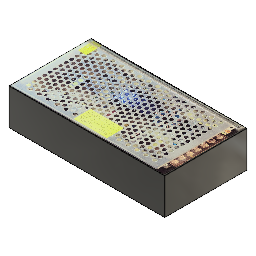
Full Assembly v14 (Autodesk Fusion 360 archive; units mm, degrees)
design "Power Supply"
Autodesk Fusion 360 part; units mm, degrees
(part 1 of 6)
sketch "Sketch1" plane through (0, 0, 0) normal (0, 0, 1) x (1, 0, 0)
  line L0 (0, 0) -> (214, 0)
  line L1 (214, 0) -> (214, 113)
  line L2 (214, 113) -> (0, 113)
  line L3 (0, 113) -> (0, 0)
  dimension "d1" = 214
  dimension "d2" = 113
  constraint horizontal L0
  constraint vertical L1
  constraint horizontal L2
  constraint vertical L3
  constraint coincident L0.start L3.end
  measures "d1" distance of L0.start L0.end
  measures "d2" distance of L0.start L2.end
extrude "Extrude1" add sketch "Sketch1" along normal blind 50

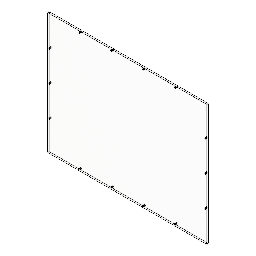
design "Front Acrylic"
Autodesk Fusion 360 part; units mm, degrees
sketch "Sketch1" plane through (0, 0, 0) normal (0, 1, 0) x (1, 0, 0)
  line L0 (0, 0) -> (635, 0)
  line L1 (635, 0) -> (635, -483.55)
  line L2 (635, -483.55) -> (0, -483.55)
  line L3 (0, -483.55) -> (0, 0)
  circle A0 centre (127, -477.05) radius 2.25
  circle A1 centre (254, -477.05) radius 2.25
  circle A2 centre (508, -477.05) radius 2.25
  circle A3 centre (381, -477.05) radius 2.25
  circle A4 centre (628.5, -362.775) radius 2.25
  circle A5 centre (628.5, -241.775) radius 2.25
  circle A6 centre (628.5, -120.775) radius 2.25
  circle A7 centre (6.5, -362.775) radius 2.25
  circle A8 centre (6.5, -241.775) radius 2.25
  circle A9 centre (6.5, -120.775) radius 2.25
  circle A10 centre (127, -6.5) radius 2.25
  circle A11 centre (254, -6.5) radius 2.25
  circle A12 centre (381, -6.5) radius 2.25
  circle A13 centre (508, -6.5) radius 2.25
  dimension "d1" = 483.55
  dimension "d2" = 635
  dimension "d5" = 6.5
  dimension "d6" = 6.5
  dimension "d7" = 127
  dimension "d8" = 127
  dimension "d9" = 127
  dimension "d10" = 127
  dimension "d11" = 6.5
  dimension "d12" = 6.5
  dimension "d13" = 6.5
  dimension "d14" = 6.5
  dimension "d15" = 6.5
  dimension "d18" = 121
  dimension "d19" = 4.5
  dimension "d21" = 121
  dimension "d22" = 121
  dimension "d23" = 6.5
  dimension "d24" = 6.5
  dimension "d26" = 6.5
  dimension "d27" = 127
  dimension "d28" = 127
  dimension "d29" = 127
  dimension "d30" = 127
  dimension "d31" = 6.5
  dimension "d32" = 6.5
  dimension "d33" = 6.5
  dimension "d34" = 6.5
  dimension "d53" = 241.775
  dimension "d54" = 121
  dimension "d55" = 241.775
  constraint horizontal L0
  constraint vertical L3
  constraint coincident L0.start L3.end
  constraint equal A0 A1
  constraint equal A1 A2
  constraint equal A2 A3
  constraint equal A3 A4
  constraint equal A4 A5
  constraint equal A5 A6
  constraint equal A0 A7
  constraint equal A7 A8
  constraint equal A8 A9
  constraint equal A10 A11
  constraint equal A11 A12
  constraint equal A12 A13
  constraint equal A9 A10
  constraint horizontal L2
  constraint vertical L1
  measures "d1" distance of L0.start L2.end
  measures "d2" distance of L0.start L0.end
  measures "d5" distance of L2 A0.centre
  measures "d6" distance of L2 A1.centre
  measures "d7" distance of L3 A0.centre
  measures "d8" distance of A0.centre A1.centre
  measures "d9" horizontal distance of A1.centre A3.centre
  measures "d10" horizontal distance of A2.centre A3.centre
  measures "d11" distance of L2 A3.centre
  measures "d12" distance of L2 A2.centre
  measures "d13" distance of L1 A4.centre
  measures "d14" distance of L1 A5.centre
  measures "d15" distance of L1 A6.centre
  measures "d18" distance of A5.centre A6.centre
  measures "d19" diameter of A0
  measures "d21" vertical distance of A7.centre A8.centre
  measures "d22" vertical distance of A8.centre A9.centre
  measures "d23" distance of L3 A7.centre
  measures "d24" distance of L3 A8.centre
  measures "d26" distance of L3 A9.centre
  measures "d27" horizontal distance of L0.start A10.centre
  measures "d28" distance of A10.centre A11.centre
  measures "d29" distance of A11.centre A12.centre
  measures "d30" distance of A12.centre A13.centre
  measures "d31" distance of L0 A10.centre
  measures "d32" distance of L0 A11.centre
  measures "d33" distance of L0 A12.centre
  measures "d34" distance of L0 A13.centre
  measures "d53" distance of L2 A5.centre
  measures "d54" distance of A4.centre A5.centre
  measures "d55" distance of L2 A8.centre
sketch "Sketch2" plane through (0, 0, 0) normal (0, 1, 0) x (1, 0, 0)
  line L0 (635, 0) -> (635, -483.55)
  line L1 (635, -483.55) -> (0, -483.55)
  line L2 (0, 0) -> (635, 0)
  line L3 (0, -483.55) -> (0, 0)
  line L4 (126, -8.5) -> (128, -8.5)
  arc A0 (128, -8.5) -> (128, -4.5) centre (128, -6.5) ccw
  line L5 (128, -4.5) -> (126, -4.5)
  arc A1 (126, -4.5) -> (126, -8.5) centre (126, -6.5) ccw
  line L6 (126, -6.5) -> (128, -6.5) construction
  line L7 (253, -8.5) -> (255, -8.5)
  arc A2 (255, -8.5) -> (255, -4.5) centre (255, -6.5) ccw
  line L8 (255, -4.5) -> (253, -4.5)
  arc A3 (253, -4.5) -> (253, -8.5) centre (253, -6.5) ccw
  line L9 (253, -6.5) -> (255, -6.5) construction
  line L10 (380, -8.5) -> (382, -8.5)
  arc A4 (382, -8.5) -> (382, -4.5) centre (382, -6.5) ccw
  line L11 (382, -4.5) -> (380, -4.5)
  arc A5 (380, -4.5) -> (380, -8.5) centre (380, -6.5) ccw
  line L12 (380, -6.5) -> (382, -6.5) construction
  line L13 (507, -8.5) -> (509, -8.5)
  arc A6 (509, -8.5) -> (509, -4.5) centre (509, -6.5) ccw
  line L14 (509, -4.5) -> (507, -4.5)
  arc A7 (507, -4.5) -> (507, -8.5) centre (507, -6.5) ccw
  line L15 (507, -6.5) -> (509, -6.5) construction
  line L16 (626.5, -119.775) -> (626.5, -121.775)
  arc A8 (626.5, -121.775) -> (630.5, -121.775) centre (628.5, -121.775) ccw
  line L17 (630.5, -121.775) -> (630.5, -119.775)
  arc A9 (630.5, -119.775) -> (626.5, -119.775) centre (628.5, -119.775) ccw
  line L18 (628.5, -119.775) -> (628.5, -121.775) construction
  line L19 (626.5, -240.775) -> (626.5, -242.775)
  arc A10 (626.5, -242.775) -> (630.5, -242.775) centre (628.5, -242.775) ccw
  line L20 (630.5, -242.775) -> (630.5, -240.775)
  arc A11 (630.5, -240.775) -> (626.5, -240.775) centre (628.5, -240.775) ccw
  line L21 (628.5, -240.775) -> (628.5, -242.775) construction
  line L22 (626.5, -361.775) -> (626.5, -363.775)
  arc A12 (626.5, -363.775) -> (630.5, -363.775) centre (628.5, -363.775) ccw
  line L23 (630.5, -363.775) -> (630.5, -361.775)
  arc A13 (630.5, -361.775) -> (626.5, -361.775) centre (628.5, -361.775) ccw
  line L24 (628.5, -361.775) -> (628.5, -363.775) construction
  line L25 (509, -475.05) -> (507, -475.05)
  arc A14 (507, -475.05) -> (507, -479.05) centre (507, -477.05) ccw
  line L26 (507, -479.05) -> (509, -479.05)
  arc A15 (509, -479.05) -> (509, -475.05) centre (509, -477.05) ccw
  line L27 (509, -477.05) -> (507, -477.05) construction
  line L28 (382, -475.05) -> (380, -475.05)
  arc A16 (380, -475.05) -> (380, -479.05) centre (380, -477.05) ccw
  line L29 (380, -479.05) -> (382, -479.05)
  arc A17 (382, -479.05) -> (382, -475.05) centre (382, -477.05) ccw
  line L30 (382, -477.05) -> (380, -477.05) construction
  line L31 (255, -475.05) -> (253, -475.05)
  arc A18 (253, -475.05) -> (253, -479.05) centre (253, -477.05) ccw
  line L32 (253, -479.05) -> (255, -479.05)
  arc A19 (255, -479.05) -> (255, -475.05) centre (255, -477.05) ccw
  line L33 (255, -477.05) -> (253, -477.05) construction
  line L34 (128, -475.05) -> (126, -475.05)
  arc A20 (126, -475.05) -> (126, -479.05) centre (126, -477.05) ccw
  line L35 (126, -479.05) -> (128, -479.05)
  arc A21 (128, -479.05) -> (128, -475.05) centre (128, -477.05) ccw
  line L36 (128, -477.05) -> (126, -477.05) construction
  line L37 (4.5, -361.775) -> (4.5, -363.775)
  arc A22 (4.5, -363.775) -> (8.5, -363.775) centre (6.5, -363.775) ccw
  line L38 (8.5, -363.775) -> (8.5, -361.775)
  arc A23 (8.5, -361.775) -> (4.5, -361.775) centre (6.5, -361.775) ccw
  line L39 (6.5, -361.775) -> (6.5, -363.775) construction
  line L40 (4.5, -240.775) -> (4.5, -242.775)
  arc A24 (4.5, -242.775) -> (8.5, -242.775) centre (6.5, -242.775) ccw
  line L41 (8.5, -242.775) -> (8.5, -240.775)
  arc A25 (8.5, -240.775) -> (4.5, -240.775) centre (6.5, -240.775) ccw
  line L42 (6.5, -240.775) -> (6.5, -242.775) construction
  line L43 (4.5, -119.775) -> (4.5, -121.775)
  arc A26 (4.5, -121.775) -> (8.5, -121.775) centre (6.5, -121.775) ccw
  line L44 (8.5, -121.775) -> (8.5, -119.775)
  arc A27 (8.5, -119.775) -> (4.5, -119.775) centre (6.5, -119.775) ccw
  line L45 (6.5, -119.775) -> (6.5, -121.775) construction
  point P0 (127, -6.5)
  point P1 (254, -6.5)
  point P2 (381, -6.5)
  point P3 (508, -6.5)
  point P4 (628.5, -120.775)
  point P5 (628.5, -241.775)
  point P6 (628.5, -362.775)
  point P7 (508, -477.05)
  point P8 (381, -477.05)
  point P9 (254, -477.05)
  point P10 (127, -477.05)
  point P11 (6.5, -362.775)
  point P12 (6.5, -241.775)
  point P13 (6.5, -120.775)
  point P14 (127, -6.5)
  point P15 (254, -6.5)
  point P16 (381, -6.5)
  point P17 (508, -6.5)
  point P18 (628.5, -120.775)
  point P19 (628.5, -241.775)
  point P20 (628.5, -362.775)
  point P21 (508, -477.05)
  point P22 (381, -477.05)
  point P23 (254, -477.05)
  point P24 (127, -477.05)
  point P25 (6.5, -362.775)
  point P26 (6.5, -241.775)
  point P27 (6.5, -120.775)
  point P28 (317.5, 0)
  dimension "d36" = 2
  dimension "d37" = 2
  dimension "d47" = 127
  dimension "d48" = 127
  dimension "d50" = 63.5
  dimension "d51" = 190.5
  dimension "d52" = 121
  constraint tangent L4 A0
  constraint tangent A0 L5
  constraint parallel L4 L5
  constraint tangent L5 A1
  constraint tangent L4 A1
  constraint horizontal L6
  constraint coincident P14 P0
  constraint midpoint L6 P14
  constraint tangent L7 A2
  constraint tangent A2 L8
  constraint parallel L7 L8
  constraint tangent L8 A3
  constraint tangent L7 A3
  constraint parallel L2 L9
  constraint coincident P15 P1
  constraint midpoint L9 P15
  constraint tangent L10 A4
  constraint tangent A4 L11
  constraint parallel L10 L11
  constraint tangent L11 A5
  constraint tangent L10 A5
  constraint parallel L2 L12
  constraint coincident P16 P2
  constraint midpoint L12 P16
  constraint tangent L13 A6
  constraint tangent A6 L14
  constraint parallel L13 L14
  constraint tangent L14 A7
  constraint tangent L13 A7
  constraint parallel L2 L15
  constraint coincident P17 P3
  constraint midpoint L15 P17
  constraint tangent L16 A8
  constraint tangent A8 L17
  constraint parallel L16 L17
  constraint tangent L17 A9
  constraint tangent L16 A9
  constraint perpendicular L13 L18
  constraint coincident P18 P4
  constraint midpoint L18 P18
  constraint tangent L19 A10
  constraint tangent A10 L20
  constraint parallel L19 L20
  constraint tangent L20 A11
  constraint tangent L19 A11
  constraint perpendicular L13 L21
  constraint coincident P19 P5
  constraint midpoint L21 P19
  constraint tangent L22 A12
  constraint tangent A12 L23
  constraint parallel L22 L23
  constraint tangent L23 A13
  constraint tangent L22 A13
  constraint parallel L19 L24
  constraint coincident P20 P6
  constraint midpoint L24 P20
  constraint tangent L25 A14
  constraint tangent A14 L26
  constraint parallel L25 L26
  constraint tangent L26 A15
  constraint tangent L25 A15
  constraint perpendicular L19 L27
  constraint coincident P21 P7
  constraint midpoint L27 P21
  constraint tangent L28 A16
  constraint tangent A16 L29
  constraint parallel L28 L29
  constraint tangent L29 A17
  constraint tangent L28 A17
  constraint parallel L1 L30
  constraint coincident P22 P8
  constraint midpoint L30 P22
  constraint tangent L31 A18
  constraint tangent A18 L32
  constraint parallel L31 L32
  constraint tangent L32 A19
  constraint tangent L31 A19
  constraint parallel L1 L33
  constraint coincident P23 P9
  constraint midpoint L33 P23
  constraint tangent L34 A20
  constraint tangent A20 L35
  constraint parallel L34 L35
  constraint tangent L35 A21
  constraint tangent L34 A21
  constraint parallel L1 L36
  constraint coincident P24 P10
  constraint midpoint L36 P24
  constraint tangent L37 A22
  constraint tangent A22 L38
  constraint parallel L37 L38
  constraint tangent L38 A23
  constraint tangent L37 A23
  constraint vertical L39
  constraint coincident P25 P11
  constraint midpoint L39 P25
  constraint tangent L40 A24
  constraint tangent A24 L41
  constraint parallel L40 L41
  constraint tangent L41 A25
  constraint tangent L40 A25
  constraint perpendicular L1 L42
  constraint coincident P26 P12
  constraint midpoint L42 P26
  constraint tangent L43 A26
  constraint tangent A26 L44
  constraint parallel L43 L44
  constraint tangent L44 A27
  constraint tangent L43 A27
  constraint parallel L3 L45
  constraint coincident P27 P13
  constraint midpoint L45 P27
  constraint equal A0 A3
  constraint equal L6 L9
  constraint equal A2 A5
  constraint equal L9 L12
  constraint equal A4 A7
  constraint equal L12 L15
  constraint equal A6 A9
  constraint equal L15 L18
  constraint equal A8 A11
  constraint equal L18 L21
  constraint equal L21 L24
  constraint equal A10 A13
  constraint equal A12 A15
  constraint equal L24 L27
  constraint equal A14 A17
  constraint equal L27 L30
  constraint equal A16 A19
  constraint equal L30 L33
  constraint equal A18 A21
  constraint equal L33 L36
  constraint equal A20 A22
  constraint equal L36 L39
  constraint equal A23 A24
  constraint equal L39 L42
  constraint equal A25 A26
  constraint equal L42 L45
  constraint midpoint L2 P28
  measures "d36" radius of A0
  measures "d37" distance of A1.centre A0.centre
  measures "d47" distance of P16 P17
  measures "d48" distance of P15 P16
  measures "d50" horizontal distance of P15 P28
  measures "d51" horizontal distance of P14 P28
  measures "d52" distance of P26 P27
sketch "Sketch3" plane through (0, 0, 0) normal (0, 1, 0) x (1, 0, 0)
  arc A0 (128, -8.5) -> (128, -4.5) centre (128, -6.5) ccw
  line L0 (126, -8.5) -> (128, -8.5)
  arc A1 (126, -4.5) -> (126, -8.5) centre (126, -6.5) ccw
  line L1 (128, -4.5) -> (126, -4.5)
  line L2 (116, -13) -> (138, -13)
  line L3 (138, -13) -> (138, 0)
  line L4 (138, 0) -> (116, 0)
  line L5 (116, 0) -> (116, -13)
  point P0 (126, -6.5)
  point P1 (127, -6.5)
  point P2 (128, -6.5)
  dimension "d42" = 10
  dimension "d43" = 10
  dimension "d44" = 6.5
  dimension "d45" = 6.5
  dimension "d46" = 6.5
  constraint horizontal L2
  constraint vertical L3
  constraint horizontal L4
  constraint vertical L5
  measures "d42" distance of P2 L3
  measures "d43" distance of P0 L5
  measures "d44" vertical distance of origin P1
  measures "d45" distance of P1 L4
  measures "d46" distance of P1 L2
extrude "Extrude2" add sketch "Sketch2" along normal blind 6.35
equation "d5 = ( 13 / 2 ) * 1 mm"
equation "d6 = d5"
equation "d7 = d2 / 5"
equation "d8 = d7"
equation "d9 = d8"
equation "d10 = d7"
equation "d11 = d5"
equation "d12 = d5"
equation "d13 = d5"
equation "d14 = d5"
equation "d15 = d5"
equation "d16 = d1 / 4"
equation "d18 = d54"
equation "d20 = d1 / 4"
equation "d21 = d54"
equation "d22 = d54"
equation "d23 = d5"
equation "d24 = d5"
equation "d26 = d5"
equation "d27 = d2 / 5"
equation "d28 = d27"
equation "d29 = d27"
equation "d30 = d27"
equation "d31 = d5"
equation "d32 = d5"
equation "d33 = d5"
equation "d34 = d5"
equation "d36 = ( 4 / 2 ) * 1 mm"
equation "d45 = d44"
equation "d46 = d44"
equation "d53 = d1 / 2"
equation "d55 = d1 / 2"

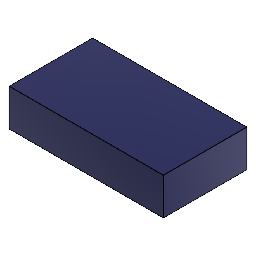
design "Power Distribution Board"
Autodesk Fusion 360 part; units mm, degrees
sketch "Sketch1" plane through (0, 0, 0) normal (0, 0, 1) x (1, 0, 0)
  line L0 (0, 0) -> (83.05, 0)
  line L1 (83.05, 0) -> (83.05, 44.95)
  line L2 (83.05, 44.95) -> (0, 44.95)
  line L3 (0, 44.95) -> (0, 0)
  dimension "d1" = 83.05
  dimension "d2" = 44.95
  constraint horizontal L0
  constraint vertical L1
  constraint horizontal L2
  constraint vertical L3
  constraint coincident L0.start L3.end
  measures "d1" distance of L0.start L0.end
  measures "d2" distance of L0.start L2.end
extrude "Extrude1" add sketch "Sketch1" along normal blind 20
equation "d1 = 82.55 mm + 0.5 mm"

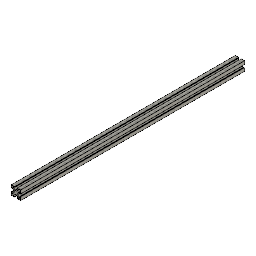
design "TS10-10"
Autodesk Fusion 360 part; units mm, degrees
sketch "Sketch1" plane through (0, 0, 0) normal (0, 1, 0) x (1, 0, 0)
  line L0 (0, 0) -> (0, 4.826)
  line L1 (0, 4.826) -> (2, 4.826)
  line L2 (2, 4.826) -> (7.874, 10.7)
  line L3 (7.874, 10.7) -> (3.302, 10.7)
  line L4 (3.302, 10.7) -> (3.302, 12.7)
  line L5 (3.302, 12.7) -> (12.7, 12.7)
  line L6 (12.7, 12.7) -> (12.7, 3.302)
  line L7 (12.7, 3.302) -> (10.7, 3.302)
  line L8 (10.7, 3.302) -> (10.7, 7.874)
  line L9 (10.7, 7.874) -> (4.826, 2)
  line L10 (4.826, 2) -> (4.826, 0)
  line L11 (4.826, 0) -> (0, 0)
  line L12 (0, 4.826) -> (-2, 4.826)
  line L13 (-4.826, 2) -> (-4.826, 0)
  line L14 (-7.874, 10.7) -> (-3.302, 10.7)
  line L15 (-10.7, 3.302) -> (-10.7, 7.874)
  line L16 (-4.826, 0) -> (0, 0)
  line L17 (-12.7, 3.302) -> (-10.7, 3.302)
  line L18 (-3.302, 10.7) -> (-3.302, 12.7)
  line L19 (-2, 4.826) -> (-7.874, 10.7)
  line L20 (-12.7, 12.7) -> (-12.7, 3.302)
  line L21 (-3.302, 12.7) -> (-12.7, 12.7)
  line L22 (-10.7, 7.874) -> (-4.826, 2)
  line L23 (0, -4.826) -> (2, -4.826)
  line L24 (12.7, -3.302) -> (10.7, -3.302)
  line L25 (7.874, -10.7) -> (3.302, -10.7)
  line L26 (3.302, -10.7) -> (3.302, -12.7)
  line L27 (3.302, -12.7) -> (12.7, -12.7)
  line L28 (-12.7, -3.302) -> (-10.7, -3.302)
  line L29 (10.7, -7.874) -> (4.826, -2)
  line L30 (-10.7, -7.874) -> (-4.826, -2)
  line L31 (-10.7, -3.302) -> (-10.7, -7.874)
  line L32 (-12.7, -12.7) -> (-12.7, -3.302)
  line L33 (12.7, -12.7) -> (12.7, -3.302)
  line L34 (4.826, -2) -> (4.826, 0)
  line L35 (2, -4.826) -> (7.874, -10.7)
  line L36 (10.7, -3.302) -> (10.7, -7.874)
  line L37 (0, -4.826) -> (-2, -4.826)
  line L38 (-7.874, -10.7) -> (-3.302, -10.7)
  line L39 (-4.826, -2) -> (-4.826, 0)
  line L40 (-3.302, -10.7) -> (-3.302, -12.7)
  line L41 (0, 0) -> (0, -4.826)
  line L42 (-2, -4.826) -> (-7.874, -10.7)
  line L43 (-3.302, -12.7) -> (-12.7, -12.7)
  dimension "d1" = 12.7
  dimension "d2" = 12.7
  dimension "d3" = 3.302
  dimension "d4" = 3.302
  dimension "d5" = 7.874
  dimension "d6" = 7.874
  dimension "d8" = 7.874
  dimension "d9" = 2
  dimension "d10" = 2
  constraint coincident L0.start L11.end
  constraint vertical L0
  constraint perpendicular L0 L1
  constraint perpendicular L3 L4
  constraint perpendicular L4 L5
  constraint perpendicular L5 L6
  constraint perpendicular L4 L7
  constraint perpendicular L0 L11
  constraint vertical L10
  constraint coincident L3.end L4.start
  constraint coincident L7.end L8.start
  constraint vertical L8
  constraint equal L3 L8
  constraint parallel L2 L9
  constraint equal L1 L10
  constraint symmetric L11.end L0 L16.end
  constraint symmetric L1.start L0 L12.start
  constraint symmetric L0 L1.end L12.end
  constraint symmetric L0 L2.end L14.start
  constraint symmetric L0 L3.end L14.end
  constraint symmetric L0 L4.end L18.end
  constraint symmetric L0 L5.end L20.start
  constraint symmetric L0 L6.end L17.start
  constraint symmetric L0 L7.end L15.start
  constraint symmetric L0 L8.end L15.end
  constraint symmetric L0 L9.end L13.start
  constraint symmetric L0 L10.end L13.end
  constraint symmetric L0.start L11 L16.end
  constraint symmetric L0.end L11 L23.start
  constraint symmetric L1.end L11 L23.end
  constraint symmetric L2.end L11 L25.start
  constraint symmetric L3.end L11 L25.end
  constraint symmetric L4.end L11 L26.end
  constraint symmetric L5.end L11 L27.end
  constraint symmetric L6.end L11 L24.start
  constraint symmetric L7.end L11 L24.end
  constraint symmetric L8.end L11 L29.start
  constraint symmetric L9.end L11 L29.end
  constraint symmetric L10.end L11 L34.end
  constraint symmetric L11 L0.start L16.end
  constraint symmetric L11 L0.end L23.start
  constraint symmetric L11 L12.end L37.end
  constraint symmetric L11 L15.start L28.end
  constraint symmetric L11 L15.end L30.start
  constraint symmetric L11 L17.start L28.start
  constraint symmetric L11 L20.start L32.start
  constraint symmetric L11 L13.end L16.start
  constraint symmetric L11 L13.start L30.end
  constraint symmetric L11 L18.end L40.end
  constraint symmetric L11 L14.start L38.start
  constraint symmetric L11 L14.end L38.end
  measures "d1" horizontal distance of L0.start L5.end
  measures "d2" vertical distance of L0.start L5.end
  measures "d3" horizontal distance of L0.start L4.end
  measures "d4" vertical distance of L0.start L6.end
  measures "d5" distance of L1 L5
  measures "d6" distance of L6 L10
  measures "d8" horizontal distance of L0.start L2.end
  measures "d9" distance of L3.end L4.end
  measures "d10" distance of L6.end L7.end
extrude "Extrude1" add sketch "Sketch1" along normal blind 609.33
equation "d2 = d1"
equation "d3 = 0.26 in / 2"
equation "d4 = d3"
equation "d8 = 0.62 in / 2"

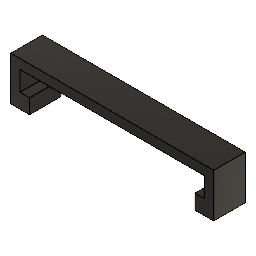
design "Bracket"
Autodesk Fusion 360 part; units mm, degrees
sketch "Sketch1" plane through (0, 0, 0) normal (0, 1, 0) x (1, 0, 0)
  line L0 (-32, 13.9) -> (-32, 0)
  line L1 (-32, 0) -> (32, 0)
  line L2 (32, 0) -> (32, 13.9)
  line L3 (32, 13.9) -> (26, 13.9)
  line L4 (29, 3) -> (-29, 3)
  line L5 (-26, 13.9) -> (-32, 13.9)
  line L6 (-29, 3) -> (-29, 9.2)
  line L7 (-29, 9.2) -> (-26, 9.2)
  line L8 (-26, 9.2) -> (-26, 13.9)
  line L9 (29, 3) -> (29, 9.2)
  line L10 (29, 9.2) -> (26, 9.2)
  line L11 (26, 9.2) -> (26, 13.9)
  dimension "d2" = 3
  dimension "d3" = 3
  dimension "d4" = 4.7
  dimension "d6" = 3
  dimension "d7" = 6.2
  dimension "d8" = 58
  constraint vertical L0
  constraint perpendicular L0 L1
  constraint perpendicular L1 L2
  constraint perpendicular L2 L4
  constraint horizontal L3
  constraint horizontal L5
  constraint collinear L3 L5
  constraint equal L3 L5
  constraint midpoint origin L1
  constraint perpendicular L4 L6
  constraint perpendicular L6 L7
  constraint perpendicular L4 L8
  constraint perpendicular L4 L9
  constraint perpendicular L9 L10
  constraint perpendicular L10 L11
  constraint collinear L7 L10
  constraint equal L7 L10
  measures "d2" distance of L0 L6
  measures "d3" distance of L1 L4
  measures "d4" distance of L7.end L5.start
  measures "d6" distance of L6.end L7.end
  measures "d7" distance of L4 L7
  measures "d8" distance of L4.start L4.end
extrude "Extrude1" add sketch "Sketch1" along normal blind 10
equation "d3 = d2"

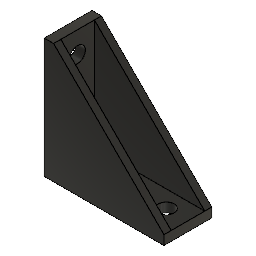
design "Small Bracket"
Autodesk Fusion 360 part; units mm, degrees
sketch "Sketch1" plane through (0, 0, 0) normal (0, 1, 0) x (1, 0, 0)
  line L0 (0, 0) -> (50, 0)
  line L1 (50, 0) -> (50, -4)
  line L2 (50, -4) -> (4, -4)
  line L3 (4, -4) -> (4, -50)
  line L4 (4, -50) -> (0, -50)
  line L5 (0, -50) -> (0, 0)
  line L6 (4, -50) -> (50, -4)
  dimension "d1" = 4
  dimension "d2" = 4
  dimension "d3" = 50
  dimension "d4" = 50
  constraint coincident L0.start L5.end
  constraint horizontal L0
  constraint perpendicular L0 L1
  constraint perpendicular L1 L2
  constraint perpendicular L2 L3
  constraint perpendicular L3 L4
  constraint perpendicular L0 L5
  measures "d1" distance of L0.end L1.end
  measures "d2" distance of L3.end L4.end
  measures "d3" distance of L4.end L0.start
  measures "d4" distance of L0.start L0.end
extrude "Extrude1" add sketch "Sketch1" along normal blind 20
extrude "Extrude2" cut sketch "Sketch1" along normal blind 17 contours L2 L3 L6
extrude "Extrude3" add sketch "Sketch1" along normal blind 3 contours L2 L3 L6
sketch "Sketch2" plane through (0, 0, 0) normal (0, 0, -1) x (1, 0, 0)
  line L0 (50, 0) -> (0, 0)
  line L1 (0, 0) -> (0, -20)
  line L2 (0, -20) -> (50, -20)
  line L3 (50, -20) -> (50, 0)
  point P0 (15, -10)
  point P1 (41, -10)
  dimension "d12" = 20
  dimension "d13" = 10
  dimension "d14" = 10
  dimension "d24" = 26
  dimension "d25" = 15
  measures "d12" distance of L0.end L1.end
  measures "d13" vertical distance of L0.end P0
  measures "d14" vertical distance of L0.end P1
  measures "d24" distance of P0 P1
  measures "d25" horizontal distance of L0.end P0
hole "Hole1" at (15, 10, 0) at (41, 10, 0) direction (0, 0, 1) diameter 6.5 depth 11 tip angle 180
sketch "Sketch3" plane through (0, 0, 0) normal (-1, 0, 0) x (0, -1, 0)
  line L0 (0, 0) -> (0, 50)
  line L1 (0, 50) -> (-20, 50)
  line L2 (-20, 50) -> (-20, 0)
  line L3 (-20, 0) -> (0, 0)
  point P0 (-10, 15)
  point P1 (-10, 41)
  dimension "d19" = 15
  dimension "d26" = 26
  measures "d19" vertical distance of L0.start P0
  measures "d26" distance of P0 P1
hole "Hole2" at (0, 10, 15) at (0, 10, 41) direction (1, 0, 0) diameter 6.5 depth 11 tip angle 180
equation "d13 = d12 / 2"
equation "d14 = d12 / 2"

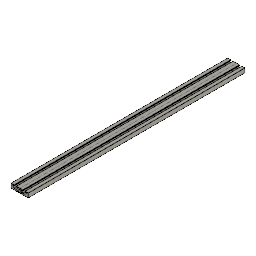
design "TS20-50-635"
Autodesk Fusion 360 part; units mm, degrees
sketch "Sketch1" plane through (0, 0, 0) normal (0, 1, 0) x (1, 0, 0)
  line L0 (0, 0) -> (25.4, 0)
  line L1 (-6.6089, -2) -> (0, -10.7)
  line L2 (9.398, -10.2) -> (9.398, -12.7)
  line L3 (-20.1422, -10.2) -> (-16.002, -4.7498)
  line L4 (25.4, -12.7) -> (16.002, -12.7)
  line L5 (-9.398, -10.2) -> (-9.398, -12.7)
  line L6 (-16.002, -12.7) -> (-16.002, -10.2)
  line L7 (0, 0) -> (0, -2)
  line L8 (9.398, -4.7498) -> (5.2578, -10.2)
  line L9 (16.002, -12.7) -> (16.002, -10.2)
  line L10 (0, 0) -> (-25.4, 0)
  line L11 (-5.2578, -10.2) -> (-9.398, -10.2)
  line L12 (-25.4, -12.7) -> (-16.002, -12.7)
  line L13 (-25.4, 0) -> (-25.4, -12.7)
  line L14 (0, -2) -> (6.6089, -2)
  line L15 (6.6089, -2) -> (0, -10.7)
  line L16 (-16.002, -10.2) -> (-20.1422, -10.2)
  line L17 (-9.398, -12.7) -> (0, -12.7)
  line L18 (0, -2) -> (-6.6089, -2)
  line L19 (-16.002, -4.7498) -> (-9.398, -4.7498)
  line L20 (16.002, -10.2) -> (20.1422, -10.2)
  line L21 (25.4, 0) -> (25.4, -12.7)
  line L22 (9.398, -12.7) -> (0, -12.7)
  line L23 (5.2578, -10.2) -> (9.398, -10.2)
  line L24 (20.1422, -10.2) -> (16.002, -4.7498)
  line L25 (16.002, -4.7498) -> (9.398, -4.7498)
  line L26 (-9.398, -4.7498) -> (-5.2578, -10.2)
  line L27 (0, -10.7) -> (0, -12.7)
  dimension "d1" = 12.7
  dimension "d2" = 2.5
  dimension "d3" = 6.604
  dimension "d4" = 6.604
  dimension "d5" = 14.8844
  dimension "d6" = 7.9502
  dimension "d7" = 25.4
  dimension "d8" = 9.398
  dimension "d9" = 2
  dimension "d10" = 2
  constraint horizontal L10
  constraint perpendicular L10 L13
  constraint perpendicular L12 L13
  constraint perpendicular L6 L12
  constraint perpendicular L6 L16
  constraint perpendicular L6 L19
  constraint parallel L11 L19
  constraint perpendicular L5 L11
  constraint perpendicular L5 L17
  constraint collinear L12 L17
  constraint collinear L11 L16
  constraint equal L11 L16
  constraint collinear L19.end L5.end L5.start
  constraint coincident L0.start L7.start
  constraint perpendicular L7 L17
  constraint perpendicular L7 L18
  constraint coincident L1.end L7
  constraint parallel L1 L26
  constraint collinear L7 L27
  constraint symmetric L0.start L10.start L7
  constraint symmetric L0.end L10.end L7
  constraint symmetric L4.start L12.start L7
  constraint symmetric L4.end L6.start L7
  constraint symmetric L9.end L6.end L7
  constraint symmetric L20.end L3.start L7
  constraint symmetric L24.end L3.end L7
  constraint symmetric L8.start L19.end L7
  constraint symmetric L8.end L11.start L7
  constraint symmetric L2.start L5.start L7
  constraint symmetric L2.end L5.end L7
  constraint symmetric L17.end L22.end L7
  constraint symmetric L14.start L18.start L7
  constraint symmetric L1.start L14.end L7
  constraint symmetric L1.end L15.end L7
  measures "d1" distance of L10 L12
  measures "d2" distance of L12 L16
  measures "d3" distance of L6.start L5.end
  measures "d4" distance of L3.end L19.end
  measures "d5" distance of L3.start L11.start
  measures "d6" vertical distance of L3.end L6.start
  measures "d7" distance of L0.start L13
  measures "d8" horizontal distance of L0.start L5.end
  measures "d9" distance of L7.end L0.start
  measures "d10" distance of L17.end L1.end
extrude "Extrude1" add sketch "Sketch1" along normal blind 635.4 contours L0 L2 L4 L7 L8 L9 L14 L15 L20 L21 L22 L23 L24 L25 L27 | L1 L3 L5 L6 L7 L10 L11 L12 L13 L16 L17 L18 L19 L26 L27
equation "d8 = d7 / 2 - d3 / 2"
equation "d11 = 610 mm + 12.7 mm * 2"

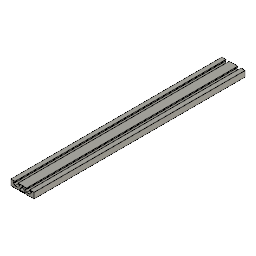
design "TS20-50-459"
Autodesk Fusion 360 part; units mm, degrees
sketch "Sketch1" plane through (0, 0, 0) normal (0, 1, 0) x (1, 0, 0)
  line L0 (0, 0) -> (-25.4, 0)
  line L1 (-25.4, 0) -> (-25.4, -12.7)
  line L2 (-25.4, -12.7) -> (-16.002, -12.7)
  line L3 (-16.002, -12.7) -> (-16.002, -10.2)
  line L4 (-16.002, -10.2) -> (-20.1422, -10.2)
  line L5 (-20.1422, -10.2) -> (-16.002, -4.7498)
  line L6 (-16.002, -4.7498) -> (-9.398, -4.7498)
  line L7 (-9.398, -4.7498) -> (-5.2578, -10.2)
  line L8 (-5.2578, -10.2) -> (-9.398, -10.2)
  line L9 (-9.398, -10.2) -> (-9.398, -12.7)
  line L10 (-9.398, -12.7) -> (0, -12.7)
  line L11 (0, -2) -> (-6.6089, -2)
  line L12 (-6.6089, -2) -> (0, -10.7)
  line L13 (0, 0) -> (0, -2)
  line L14 (0, -10.7) -> (0, -12.7)
  line L15 (9.398, -10.2) -> (9.398, -12.7)
  line L16 (16.002, -4.7498) -> (9.398, -4.7498)
  line L17 (16.002, -12.7) -> (16.002, -10.2)
  line L18 (5.2578, -10.2) -> (9.398, -10.2)
  line L19 (20.1422, -10.2) -> (16.002, -4.7498)
  line L20 (25.4, 0) -> (25.4, -12.7)
  line L21 (9.398, -12.7) -> (0, -12.7)
  line L22 (16.002, -10.2) -> (20.1422, -10.2)
  line L23 (0, 0) -> (25.4, 0)
  line L24 (6.6089, -2) -> (0, -10.7)
  line L25 (9.398, -4.7498) -> (5.2578, -10.2)
  line L26 (0, -2) -> (6.6089, -2)
  line L27 (25.4, -12.7) -> (16.002, -12.7)
  dimension "d1" = 12.7
  dimension "d2" = 2.5
  dimension "d3" = 6.604
  dimension "d4" = 6.604
  dimension "d5" = 14.8844
  dimension "d6" = 7.9502
  dimension "d7" = 25.4
  dimension "d8" = 9.398
  dimension "d9" = 2
  dimension "d10" = 2
  constraint horizontal L0
  constraint perpendicular L0 L1
  constraint perpendicular L1 L2
  constraint perpendicular L2 L3
  constraint perpendicular L3 L4
  constraint perpendicular L3 L6
  constraint parallel L6 L8
  constraint perpendicular L8 L9
  constraint perpendicular L9 L10
  constraint collinear L2 L10
  constraint collinear L4 L8
  constraint equal L4 L8
  constraint collinear L6.end L8.end L9.end
  constraint coincident L0.start L13.start
  constraint perpendicular L10 L13
  constraint perpendicular L11 L13
  constraint coincident L12.end L13
  constraint parallel L7 L12
  constraint collinear L13 L14
  constraint symmetric L0.start L13 L23.start
  constraint symmetric L0.end L13 L20.start
  constraint symmetric L1.end L13 L20.end
  constraint symmetric L2.end L13 L17.start
  constraint symmetric L3.end L13 L17.end
  constraint symmetric L4.end L13 L19.start
  constraint symmetric L5.end L13 L16.start
  constraint symmetric L6.end L13 L16.end
  constraint symmetric L7.end L13 L18.start
  constraint symmetric L8.end L13 L15.start
  constraint symmetric L9.end L13 L15.end
  constraint symmetric L10.end L13 L14.end
  constraint symmetric L11.start L13 L26.start
  constraint symmetric L11.end L13 L24.start
  constraint symmetric L12.end L13 L14.start
  measures "d1" distance of L0 L2
  measures "d2" distance of L2 L4
  measures "d3" distance of L2.end L9.end
  measures "d4" distance of L5.end L6.end
  measures "d5" distance of L4.end L7.end
  measures "d6" vertical distance of L2.end L5.end
  measures "d7" distance of L0.start L1
  measures "d8" horizontal distance of L0.start L9.end
  measures "d9" distance of L0.start L11.start
  measures "d10" distance of L10.end L12.end
extrude "Extrude1" add sketch "Sketch1" along normal blind 459 contours L0 L1 L2 L3 L4 L5 L6 L7 L8 L9 L10 L11 L12 L13 L14 | L13 L14 L15 L16 L17 L18 L19 L20 L21 L22 L23 L24 L25 L26 L27
equation "d8 = d7 / 2 - d3 / 2"

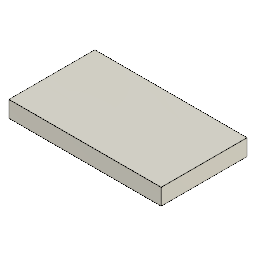
design "Single Panel"
Autodesk Fusion 360 part; units mm, degrees
sketch "Sketch1" plane through (0, 0, 0) normal (0, 0, 1) x (1, 0, 0)
  line L0 (0, 0) -> (203.3333, 0)
  line L1 (203.3333, 0) -> (203.3333, 114.75)
  line L2 (203.3333, 114.75) -> (0, 114.75)
  line L3 (0, 114.75) -> (0, 0)
  dimension "d1" = 203.3333
  dimension "d2" = 114.75
  constraint horizontal L0
  constraint vertical L1
  constraint horizontal L2
  constraint vertical L3
  constraint coincident L0.start L3.end
  measures "d1" distance of L0.start L0.end
  measures "d2" distance of L0.start L2.end
extrude "Extrude1" add sketch "Sketch1" along normal blind 22
sketch "Sketch2" plane through (0, 0, 0) normal (0, 0, 1) x (1, 0, 0)
  line L0 (0, 0) -> (12.7083, 0)
  line L1 (12.7083, 0) -> (12.7083, 19.125)
  line L2 (12.7083, 19.125) -> (0, 19.125)
  line L3 (0, 19.125) -> (0, 0)
  line L4 (0, 0) -> (203.3333, 0)
  line L5 (0, 114.75) -> (0, 0)
  line L6 (9.2083, 16.625) -> (10.1943, 9.6615)
  line L7 (10.1943, 9.6615) -> (9.4443, 9.6615)
  line L8 (9.4443, 9.6615) -> (8.5483, 10.5871)
  line L9 (8.5483, 10.5871) -> (7.6934, 16.625)
  line L10 (7.6934, 16.625) -> (9.2083, 16.625)
  line L11 (7.4934, 16.625) -> (7.7058, 15.125)
  line L12 (7.7058, 15.125) -> (3.4274, 15.125)
  line L13 (3.4274, 15.125) -> (3.215, 16.625)
  line L14 (3.215, 16.625) -> (7.4934, 16.625)
  line L15 (9.274, 9.5499) -> (8.5357, 10.3126)
  line L16 (8.5357, 10.3126) -> (4.1969, 10.3126)
  line L17 (4.1969, 10.3126) -> (3.4334, 9.5752)
  line L18 (3.4334, 9.5752) -> (4.1717, 8.8126)
  line L19 (4.1717, 8.8126) -> (8.5104, 8.8126)
  line L20 (8.5104, 8.8126) -> (9.274, 9.5499)
  line L21 (10.2224, 9.4635) -> (9.4724, 9.4635)
  line L22 (9.4724, 9.4635) -> (8.8126, 8.8263)
  line L23 (8.8126, 8.8263) -> (9.7083, 2.5)
  line L24 (9.7083, 2.5) -> (11.2083, 2.5)
  line L25 (11.2083, 2.5) -> (10.2224, 9.4635)
  line L26 (9.5063, 2.5) -> (9.2939, 4)
  line L27 (9.2939, 4) -> (5.0046, 4)
  line L28 (5.0046, 4) -> (5.217, 2.5)
  line L29 (5.217, 2.5) -> (9.5063, 2.5)
  line L30 (5.015, 2.5) -> (3.5, 2.5)
  line L31 (3.5, 2.5) -> (2.5142, 9.4625)
  line L32 (2.5142, 9.4625) -> (3.2642, 9.4625)
  line L33 (3.2642, 9.4625) -> (4.1602, 8.5369)
  line L34 (4.1602, 8.5369) -> (5.015, 2.5)
  line L35 (3.015, 16.625) -> (3.9088, 10.3124)
  line L36 (3.9088, 10.3124) -> (3.2358, 9.6625)
  line L37 (3.2358, 9.6625) -> (2.4858, 9.6625)
  line L38 (2.4858, 9.6625) -> (1.5, 16.625)
  line L39 (3.015, 16.625) -> (1.5, 16.625)
  circle A0 centre (1.5, 3.375) radius 0.875
  arc A1 (10.6325, 2.5) -> (11.1276, 3.0701) centre (10.6325, 3) ccw
  arc A2 (9.2692, 16.1951) -> (8.7741, 16.625) centre (8.7741, 16.125) ccw
  arc A3 (2.0758, 16.625) -> (1.5807, 16.0549) centre (2.0758, 16.125) ccw
  arc A4 (3.4391, 2.9299) -> (3.9342, 2.5) centre (3.9342, 3) ccw
  line L40 (20.4138, 15.125) -> (16.1354, 15.125)
  line L41 (15.723, 16.625) -> (14.208, 16.625)
  arc A5 (23.3405, 2.5) -> (23.8356, 3.0701) centre (23.3405, 3) ccw
  circle A6 centre (14.208, 3.375) radius 0.875
  line L42 (15.9722, 9.4625) -> (16.8682, 8.5369)
  line L43 (22.4163, 2.5) -> (23.9163, 2.5)
  line L44 (22.0019, 4) -> (17.7126, 4)
  line L45 (16.9049, 10.3126) -> (16.1414, 9.5752)
  line L46 (17.723, 2.5) -> (16.208, 2.5)
  line L47 (16.208, 2.5) -> (15.2222, 9.4625)
  line L48 (21.5206, 8.8263) -> (22.4163, 2.5)
  line L49 (22.2143, 2.5) -> (22.0019, 4)
  line L50 (21.2184, 8.8126) -> (21.982, 9.5499)
  line L51 (22.9023, 9.6615) -> (22.1523, 9.6615)
  line L52 (23.9163, 2.5) -> (22.9304, 9.4635)
  arc A7 (14.7838, 16.625) -> (14.2887, 16.0549) centre (14.7838, 16.125) ccw
  line L53 (17.925, 2.5) -> (22.2143, 2.5)
  line L54 (16.8682, 8.5369) -> (17.723, 2.5)
  line L55 (22.1804, 9.4635) -> (21.5206, 8.8263)
  line L56 (17.7126, 4) -> (17.925, 2.5)
  line L57 (16.8797, 8.8126) -> (21.2184, 8.8126)
  line L58 (22.1523, 9.6615) -> (21.2563, 10.5871)
  line L59 (15.2222, 9.4625) -> (15.9722, 9.4625)
  line L60 (22.9304, 9.4635) -> (22.1804, 9.4635)
  arc A8 (16.1471, 2.9299) -> (16.6422, 2.5) centre (16.6422, 3) ccw
  line L61 (15.9438, 9.6625) -> (15.1938, 9.6625)
  line L62 (20.2014, 16.625) -> (20.4138, 15.125)
  arc A9 (21.9772, 16.1951) -> (21.4821, 16.625) centre (21.4821, 16.125) ccw
  line L63 (15.1938, 9.6625) -> (14.208, 16.625)
  line L64 (16.1354, 15.125) -> (15.923, 16.625)
  line L65 (21.9163, 16.625) -> (22.9023, 9.6615)
  line L66 (16.1414, 9.5752) -> (16.8797, 8.8126)
  line L67 (15.723, 16.625) -> (16.6168, 10.3124)
  line L68 (21.982, 9.5499) -> (21.2437, 10.3126)
  line L69 (21.2563, 10.5871) -> (20.4014, 16.625)
  line L70 (15.923, 16.625) -> (20.2014, 16.625)
  line L71 (21.2437, 10.3126) -> (16.9049, 10.3126)
  line L72 (20.4014, 16.625) -> (21.9163, 16.625)
  line L73 (16.6168, 10.3124) -> (15.9438, 9.6625)
  line L74 (33.1218, 15.125) -> (28.8434, 15.125)
  line L75 (28.431, 16.625) -> (26.916, 16.625)
  arc A10 (36.0485, 2.5) -> (36.5436, 3.0701) centre (36.0485, 3) ccw
  circle A11 centre (26.916, 3.375) radius 0.875
  line L76 (28.6802, 9.4625) -> (29.5762, 8.5369)
  line L77 (35.1243, 2.5) -> (36.6243, 2.5)
  line L78 (34.7099, 4) -> (30.4206, 4)
  line L79 (29.6129, 10.3126) -> (28.8494, 9.5752)
  line L80 (30.431, 2.5) -> (28.916, 2.5)
  line L81 (28.916, 2.5) -> (27.9302, 9.4625)
  line L82 (34.2286, 8.8263) -> (35.1243, 2.5)
  line L83 (34.9223, 2.5) -> (34.7099, 4)
  line L84 (33.9264, 8.8126) -> (34.69, 9.5499)
  line L85 (35.6103, 9.6615) -> (34.8603, 9.6615)
  line L86 (36.6243, 2.5) -> (35.6384, 9.4635)
  arc A12 (27.4918, 16.625) -> (26.9967, 16.0549) centre (27.4918, 16.125) ccw
  line L87 (30.633, 2.5) -> (34.9223, 2.5)
  line L88 (29.5762, 8.5369) -> (30.431, 2.5)
  line L89 (34.8884, 9.4635) -> (34.2286, 8.8263)
  line L90 (30.4206, 4) -> (30.633, 2.5)
  line L91 (29.5877, 8.8126) -> (33.9264, 8.8126)
  line L92 (34.8603, 9.6615) -> (33.9643, 10.5871)
  line L93 (27.9302, 9.4625) -> (28.6802, 9.4625)
  line L94 (35.6384, 9.4635) -> (34.8884, 9.4635)
  arc A13 (28.8551, 2.9299) -> (29.3502, 2.5) centre (29.3502, 3) ccw
  line L95 (28.6518, 9.6625) -> (27.9018, 9.6625)
  line L96 (32.9094, 16.625) -> (33.1218, 15.125)
  arc A14 (34.6852, 16.1951) -> (34.1901, 16.625) centre (34.1901, 16.125) ccw
  line L97 (27.9018, 9.6625) -> (26.916, 16.625)
  line L98 (28.8434, 15.125) -> (28.631, 16.625)
  line L99 (34.6243, 16.625) -> (35.6103, 9.6615)
  line L100 (28.8494, 9.5752) -> (29.5877, 8.8126)
  line L101 (28.431, 16.625) -> (29.3248, 10.3124)
  line L102 (34.69, 9.5499) -> (33.9517, 10.3126)
  line L103 (33.9643, 10.5871) -> (33.1094, 16.625)
  line L104 (28.631, 16.625) -> (32.9094, 16.625)
  line L105 (33.9517, 10.3126) -> (29.6129, 10.3126)
  line L106 (33.1094, 16.625) -> (34.6243, 16.625)
  line L107 (29.3248, 10.3124) -> (28.6518, 9.6625)
  line L108 (45.8298, 15.125) -> (41.5514, 15.125)
  line L109 (41.139, 16.625) -> (39.624, 16.625)
  arc A15 (48.7565, 2.5) -> (49.2516, 3.0701) centre (48.7565, 3) ccw
  circle A16 centre (39.624, 3.375) radius 0.875
  line L110 (41.3882, 9.4625) -> (42.2842, 8.5369)
  line L111 (47.8323, 2.5) -> (49.3323, 2.5)
  line L112 (47.4179, 4) -> (43.1286, 4)
  line L113 (42.3209, 10.3126) -> (41.5574, 9.5752)
  line L114 (43.139, 2.5) -> (41.624, 2.5)
  line L115 (41.624, 2.5) -> (40.6382, 9.4625)
  line L116 (46.9366, 8.8263) -> (47.8323, 2.5)
  line L117 (47.6303, 2.5) -> (47.4179, 4)
  line L118 (46.6344, 8.8126) -> (47.398, 9.5499)
  line L119 (48.3183, 9.6615) -> (47.5683, 9.6615)
  line L120 (49.3323, 2.5) -> (48.3464, 9.4635)
  arc A17 (40.1998, 16.625) -> (39.7047, 16.0549) centre (40.1998, 16.125) ccw
  line L121 (43.341, 2.5) -> (47.6303, 2.5)
  line L122 (42.2842, 8.5369) -> (43.139, 2.5)
  line L123 (47.5964, 9.4635) -> (46.9366, 8.8263)
  line L124 (43.1286, 4) -> (43.341, 2.5)
  line L125 (42.2957, 8.8126) -> (46.6344, 8.8126)
  line L126 (47.5683, 9.6615) -> (46.6723, 10.5871)
  line L127 (40.6382, 9.4625) -> (41.3882, 9.4625)
  line L128 (48.3464, 9.4635) -> (47.5964, 9.4635)
  arc A18 (41.5631, 2.9299) -> (42.0582, 2.5) centre (42.0582, 3) ccw
  line L129 (41.3598, 9.6625) -> (40.6098, 9.6625)
  line L130 (45.6174, 16.625) -> (45.8298, 15.125)
  arc A19 (47.3932, 16.1951) -> (46.8981, 16.625) centre (46.8981, 16.125) ccw
  line L131 (40.6098, 9.6625) -> (39.624, 16.625)
  line L132 (41.5514, 15.125) -> (41.339, 16.625)
  line L133 (47.3323, 16.625) -> (48.3183, 9.6615)
  line L134 (41.5574, 9.5752) -> (42.2957, 8.8126)
  line L135 (41.139, 16.625) -> (42.0328, 10.3124)
  line L136 (47.398, 9.5499) -> (46.6597, 10.3126)
  line L137 (46.6723, 10.5871) -> (45.8174, 16.625)
  line L138 (41.339, 16.625) -> (45.6174, 16.625)
  line L139 (46.6597, 10.3126) -> (42.3209, 10.3126)
  line L140 (45.8174, 16.625) -> (47.3323, 16.625)
  line L141 (42.0328, 10.3124) -> (41.3598, 9.6625)
  line L142 (58.5378, 15.125) -> (54.2594, 15.125)
  line L143 (53.847, 16.625) -> (52.332, 16.625)
  arc A20 (61.4645, 2.5) -> (61.9596, 3.0701) centre (61.4645, 3) ccw
  circle A21 centre (52.332, 3.375) radius 0.875
  line L144 (54.0962, 9.4625) -> (54.9922, 8.5369)
  line L145 (60.5403, 2.5) -> (62.0403, 2.5)
  line L146 (60.1259, 4) -> (55.8366, 4)
  line L147 (55.0289, 10.3126) -> (54.2654, 9.5752)
  line L148 (55.847, 2.5) -> (54.332, 2.5)
  line L149 (54.332, 2.5) -> (53.3462, 9.4625)
  line L150 (59.6446, 8.8263) -> (60.5403, 2.5)
  line L151 (60.3383, 2.5) -> (60.1259, 4)
  line L152 (59.3424, 8.8126) -> (60.106, 9.5499)
  line L153 (61.0263, 9.6615) -> (60.2763, 9.6615)
  line L154 (62.0403, 2.5) -> (61.0544, 9.4635)
  arc A22 (52.9078, 16.625) -> (52.4127, 16.0549) centre (52.9078, 16.125) ccw
  line L155 (56.049, 2.5) -> (60.3383, 2.5)
  line L156 (54.9922, 8.5369) -> (55.847, 2.5)
  line L157 (60.3044, 9.4635) -> (59.6446, 8.8263)
  line L158 (55.8366, 4) -> (56.049, 2.5)
  line L159 (55.0037, 8.8126) -> (59.3424, 8.8126)
  line L160 (60.2763, 9.6615) -> (59.3803, 10.5871)
  line L161 (53.3462, 9.4625) -> (54.0962, 9.4625)
  line L162 (61.0544, 9.4635) -> (60.3044, 9.4635)
  arc A23 (54.2711, 2.9299) -> (54.7662, 2.5) centre (54.7662, 3) ccw
  line L163 (54.0678, 9.6625) -> (53.3178, 9.6625)
  line L164 (58.3254, 16.625) -> (58.5378, 15.125)
  arc A24 (60.1012, 16.1951) -> (59.6061, 16.625) centre (59.6061, 16.125) ccw
  line L165 (53.3178, 9.6625) -> (52.332, 16.625)
  line L166 (54.2594, 15.125) -> (54.047, 16.625)
  line L167 (60.0403, 16.625) -> (61.0263, 9.6615)
  line L168 (54.2654, 9.5752) -> (55.0037, 8.8126)
  line L169 (53.847, 16.625) -> (54.7408, 10.3124)
  line L170 (60.106, 9.5499) -> (59.3677, 10.3126)
  line L171 (59.3803, 10.5871) -> (58.5254, 16.625)
  line L172 (54.047, 16.625) -> (58.3254, 16.625)
  line L173 (59.3677, 10.3126) -> (55.0289, 10.3126)
  line L174 (58.5254, 16.625) -> (60.0403, 16.625)
  line L175 (54.7408, 10.3124) -> (54.0678, 9.6625)
  line L176 (71.2458, 15.125) -> (66.9674, 15.125)
  line L177 (66.555, 16.625) -> (65.04, 16.625)
  arc A25 (74.1725, 2.5) -> (74.6676, 3.0701) centre (74.1725, 3) ccw
  circle A26 centre (65.04, 3.375) radius 0.875
  line L178 (66.8042, 9.4625) -> (67.7002, 8.5369)
  line L179 (73.2483, 2.5) -> (74.7483, 2.5)
  line L180 (72.8339, 4) -> (68.5446, 4)
  line L181 (67.7369, 10.3126) -> (66.9734, 9.5752)
  line L182 (68.555, 2.5) -> (67.04, 2.5)
  line L183 (67.04, 2.5) -> (66.0542, 9.4625)
  line L184 (72.3526, 8.8263) -> (73.2483, 2.5)
  line L185 (73.0463, 2.5) -> (72.8339, 4)
  line L186 (72.0504, 8.8126) -> (72.814, 9.5499)
  line L187 (73.7343, 9.6615) -> (72.9843, 9.6615)
  line L188 (74.7483, 2.5) -> (73.7624, 9.4635)
  arc A27 (65.6158, 16.625) -> (65.1207, 16.0549) centre (65.6158, 16.125) ccw
  line L189 (68.757, 2.5) -> (73.0463, 2.5)
  line L190 (67.7002, 8.5369) -> (68.555, 2.5)
  line L191 (73.0124, 9.4635) -> (72.3526, 8.8263)
  line L192 (68.5446, 4) -> (68.757, 2.5)
  line L193 (67.7117, 8.8126) -> (72.0504, 8.8126)
  line L194 (72.9843, 9.6615) -> (72.0883, 10.5871)
  line L195 (66.0542, 9.4625) -> (66.8042, 9.4625)
  line L196 (73.7624, 9.4635) -> (73.0124, 9.4635)
  arc A28 (66.9791, 2.9299) -> (67.4742, 2.5) centre (67.4742, 3) ccw
  line L197 (66.7758, 9.6625) -> (66.0258, 9.6625)
  line L198 (71.0334, 16.625) -> (71.2458, 15.125)
  arc A29 (72.8092, 16.1951) -> (72.3141, 16.625) centre (72.3141, 16.125) ccw
  line L199 (66.0258, 9.6625) -> (65.04, 16.625)
  line L200 (66.9674, 15.125) -> (66.755, 16.625)
  line L201 (72.7483, 16.625) -> (73.7343, 9.6615)
  line L202 (66.9734, 9.5752) -> (67.7117, 8.8126)
  line L203 (66.555, 16.625) -> (67.4488, 10.3124)
  line L204 (72.814, 9.5499) -> (72.0757, 10.3126)
  line L205 (72.0883, 10.5871) -> (71.2334, 16.625)
  line L206 (66.755, 16.625) -> (71.0334, 16.625)
  line L207 (72.0757, 10.3126) -> (67.7369, 10.3126)
  line L208 (71.2334, 16.625) -> (72.7483, 16.625)
  line L209 (67.4488, 10.3124) -> (66.7758, 9.6625)
  line L210 (83.9538, 15.125) -> (79.6754, 15.125)
  line L211 (79.263, 16.625) -> (77.748, 16.625)
  arc A30 (86.8805, 2.5) -> (87.3756, 3.0701) centre (86.8805, 3) ccw
  circle A31 centre (77.748, 3.375) radius 0.875
  line L212 (79.5122, 9.4625) -> (80.4082, 8.5369)
  line L213 (85.9563, 2.5) -> (87.4563, 2.5)
  line L214 (85.5419, 4) -> (81.2526, 4)
  line L215 (80.4449, 10.3126) -> (79.6814, 9.5752)
  line L216 (81.263, 2.5) -> (79.748, 2.5)
  line L217 (79.748, 2.5) -> (78.7622, 9.4625)
  line L218 (85.0606, 8.8263) -> (85.9563, 2.5)
  line L219 (85.7543, 2.5) -> (85.5419, 4)
  line L220 (84.7584, 8.8126) -> (85.522, 9.5499)
  line L221 (86.4423, 9.6615) -> (85.6923, 9.6615)
  line L222 (87.4563, 2.5) -> (86.4704, 9.4635)
  arc A32 (78.3238, 16.625) -> (77.8287, 16.0549) centre (78.3238, 16.125) ccw
  line L223 (81.465, 2.5) -> (85.7543, 2.5)
  line L224 (80.4082, 8.5369) -> (81.263, 2.5)
  line L225 (85.7204, 9.4635) -> (85.0606, 8.8263)
  line L226 (81.2526, 4) -> (81.465, 2.5)
  line L227 (80.4197, 8.8126) -> (84.7584, 8.8126)
  line L228 (85.6923, 9.6615) -> (84.7963, 10.5871)
  line L229 (78.7622, 9.4625) -> (79.5122, 9.4625)
  line L230 (86.4704, 9.4635) -> (85.7204, 9.4635)
  arc A33 (79.6871, 2.9299) -> (80.1822, 2.5) centre (80.1822, 3) ccw
  line L231 (79.4838, 9.6625) -> (78.7338, 9.6625)
  line L232 (83.7414, 16.625) -> (83.9538, 15.125)
  arc A34 (85.5172, 16.1951) -> (85.0221, 16.625) centre (85.0221, 16.125) ccw
  line L233 (78.7338, 9.6625) -> (77.748, 16.625)
  line L234 (79.6754, 15.125) -> (79.463, 16.625)
  line L235 (85.4563, 16.625) -> (86.4423, 9.6615)
  line L236 (79.6814, 9.5752) -> (80.4197, 8.8126)
  line L237 (79.263, 16.625) -> (80.1568, 10.3124)
  line L238 (85.522, 9.5499) -> (84.7837, 10.3126)
  line L239 (84.7963, 10.5871) -> (83.9414, 16.625)
  line L240 (79.463, 16.625) -> (83.7414, 16.625)
  line L241 (84.7837, 10.3126) -> (80.4449, 10.3126)
  line L242 (83.9414, 16.625) -> (85.4563, 16.625)
  line L243 (80.1568, 10.3124) -> (79.4838, 9.6625)
  line L244 (96.6618, 15.125) -> (92.3834, 15.125)
  line L245 (91.971, 16.625) -> (90.456, 16.625)
  arc A35 (99.5885, 2.5) -> (100.0836, 3.0701) centre (99.5885, 3) ccw
  circle A36 centre (90.456, 3.375) radius 0.875
  line L246 (92.2202, 9.4625) -> (93.1162, 8.5369)
  line L247 (98.6643, 2.5) -> (100.1643, 2.5)
  line L248 (98.2499, 4) -> (93.9606, 4)
  line L249 (93.1529, 10.3126) -> (92.3894, 9.5752)
  line L250 (93.971, 2.5) -> (92.456, 2.5)
  line L251 (92.456, 2.5) -> (91.4702, 9.4625)
  line L252 (97.7686, 8.8263) -> (98.6643, 2.5)
  line L253 (98.4623, 2.5) -> (98.2499, 4)
  line L254 (97.4664, 8.8126) -> (98.23, 9.5499)
  line L255 (99.1503, 9.6615) -> (98.4003, 9.6615)
  line L256 (100.1643, 2.5) -> (99.1784, 9.4635)
  arc A37 (91.0318, 16.625) -> (90.5367, 16.0549) centre (91.0318, 16.125) ccw
  line L257 (94.173, 2.5) -> (98.4623, 2.5)
  line L258 (93.1162, 8.5369) -> (93.971, 2.5)
  line L259 (98.4284, 9.4635) -> (97.7686, 8.8263)
  line L260 (93.9606, 4) -> (94.173, 2.5)
  line L261 (93.1277, 8.8126) -> (97.4664, 8.8126)
  line L262 (98.4003, 9.6615) -> (97.5043, 10.5871)
  line L263 (91.4702, 9.4625) -> (92.2202, 9.4625)
  line L264 (99.1784, 9.4635) -> (98.4284, 9.4635)
  arc A38 (92.3951, 2.9299) -> (92.8902, 2.5) centre (92.8902, 3) ccw
  line L265 (92.1918, 9.6625) -> (91.4418, 9.6625)
  line L266 (96.4494, 16.625) -> (96.6618, 15.125)
  arc A39 (98.2252, 16.1951) -> (97.7301, 16.625) centre (97.7301, 16.125) ccw
  line L267 (91.4418, 9.6625) -> (90.456, 16.625)
  line L268 (92.3834, 15.125) -> (92.171, 16.625)
  line L269 (98.1643, 16.625) -> (99.1503, 9.6615)
  line L270 (92.3894, 9.5752) -> (93.1277, 8.8126)
  line L271 (91.971, 16.625) -> (92.8648, 10.3124)
  line L272 (98.23, 9.5499) -> (97.4917, 10.3126)
  line L273 (97.5043, 10.5871) -> (96.6494, 16.625)
  line L274 (92.171, 16.625) -> (96.4494, 16.625)
  line L275 (97.4917, 10.3126) -> (93.1529, 10.3126)
  line L276 (96.6494, 16.625) -> (98.1643, 16.625)
  line L277 (92.8648, 10.3124) -> (92.1918, 9.6625)
  line L278 (109.3698, 15.125) -> (105.0914, 15.125)
  line L279 (104.679, 16.625) -> (103.164, 16.625)
  arc A40 (112.2965, 2.5) -> (112.7916, 3.0701) centre (112.2965, 3) ccw
  circle A41 centre (103.164, 3.375) radius 0.875
  line L280 (104.9282, 9.4625) -> (105.8242, 8.5369)
  line L281 (111.3723, 2.5) -> (112.8723, 2.5)
  line L282 (110.9579, 4) -> (106.6686, 4)
  line L283 (105.8609, 10.3126) -> (105.0974, 9.5752)
  line L284 (106.679, 2.5) -> (105.164, 2.5)
  line L285 (105.164, 2.5) -> (104.1782, 9.4625)
  line L286 (110.4766, 8.8263) -> (111.3723, 2.5)
  line L287 (111.1703, 2.5) -> (110.9579, 4)
  line L288 (110.1744, 8.8126) -> (110.938, 9.5499)
  line L289 (111.8583, 9.6615) -> (111.1083, 9.6615)
  line L290 (112.8723, 2.5) -> (111.8864, 9.4635)
  arc A42 (103.7398, 16.625) -> (103.2447, 16.0549) centre (103.7398, 16.125) ccw
  line L291 (106.881, 2.5) -> (111.1703, 2.5)
  line L292 (105.8242, 8.5369) -> (106.679, 2.5)
  line L293 (111.1364, 9.4635) -> (110.4766, 8.8263)
  line L294 (106.6686, 4) -> (106.881, 2.5)
  line L295 (105.8357, 8.8126) -> (110.1744, 8.8126)
  line L296 (111.1083, 9.6615) -> (110.2123, 10.5871)
  line L297 (104.1782, 9.4625) -> (104.9282, 9.4625)
  line L298 (111.8864, 9.4635) -> (111.1364, 9.4635)
  arc A43 (105.1031, 2.9299) -> (105.5982, 2.5) centre (105.5982, 3) ccw
  line L299 (104.8998, 9.6625) -> (104.1498, 9.6625)
  line L300 (109.1574, 16.625) -> (109.3698, 15.125)
  arc A44 (110.9332, 16.1951) -> (110.4381, 16.625) centre (110.4381, 16.125) ccw